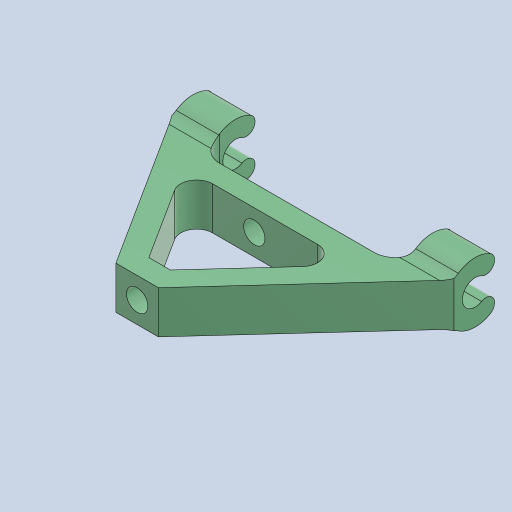
# Autodesk Inventor part: GearBase
Saved by Autodesk Inventor 2023 (Build 270158000, 158)
## iProperties
Created: 2022-06-15
Part Number: GearBase
Material: ABS プラスチック
Document SubType Name: Modeling
Designer: legot
Density: 1.06 g/cm^3
Appearance: 滑らか - 白
Mass: 0.555429 g
Surface Area: 7.58105 cm^2
Volume: 0.52399 cm^3
Author: legot
Autodesk Inventor part; units mm, degrees
ref_plane "YZ Plane" through (0, 0, 0) normal (1, 0, 0) x (0, 1, 0)
ref_plane "XZ Plane" through (0, 0, 0) normal (0, 1, 0) x (-1, 0, 0)
ref_plane "XY Plane" through (0, 0, 0) normal (0, 0, 1) x (1, 0, 0)
sketch "スケッチ1" plane through (0, 0, 0) normal (0, 1, 0) x (-1, 0, 0)
  line L0 (13.25, -2) -> (-13.25, -2)
  line L1 (-13.25, -2) -> (-13.25, 2)
  line L2 (13.25, 2) -> (13.25, -2)
  line L3 (13.25, 2) -> (4, 16.5)
  line L4 (4, 16.5) -> (0, 16.5)
  line L5 (0, 16.5) -> (-13.25, 2)
  line L6 (9.25, 3.5) -> (-9.25, 3.5)
  line L7 (9.25, 3.5) -> (9.25, -2)
  line L8 (-9.25, 3.5) -> (-9.25, -2)
  point P0 (0, 0)
  point P1 (13.25, 0)
  point P2 (0, -2)
  point P3 (2, 16.5)
  dimension "d1" = 4
  dimension "d2" = 4
  dimension "d3" = 16.5
  dimension "d19" = 3.5
  dimension "d32" = 4
  dimension "d33" = 26.5
  dimension "d34" = 4
  dimension "d36" = 4
  dimension "d37" = 2
  constraints: 18 end point, 3 horizontal, 3 midpoint, 2 parallel, 2 perpendicular, 2 point on line, 1 horizontal alignment, 1 vertical alignment
  measures "d1" distance of L2.start L0.start
  measures "d2" distance of L3.end L4.end
  measures "d3" distance from line of point (0, 0) L4
  measures "d19" distance from line of L6 point (0, 0)
  measures "d32" distance between parallel lines of L8 L1
  measures "d33" distance of L0.start L0.end
  measures "d34" distance between parallel lines of L2 L7
  measures "d36" distance of L0.end L1.end
  measures "d37" horizontal distance of point (0, -2) point (2, 16.5)
extrude "押し出し1" add sketch "スケッチ1" along normal mid plane 4 contours L0 L7 L6 L8 L1 L5 L4 L3 L2
sketch "スケッチ3" plane through (-4, 2, 16.5) normal (0, 0, 1) x (1, 0, 0)
  line L0 (0, 0) -> (4, 0) projected
  line L1 (0, -4) -> (0, 0) projected
  point P0 (4, -2)
  point P1 (2, -2)
  point P2 (0, -2)
  point P3 (2, 0)
  constraints: 2 midpoint, 1 horizontal alignment, 1 vertical alignment
hole "穴1" at (-2, 0, 16.5) direction (0, 0, -1) diameter 2 end through all
sketch "スケッチ4" plane through (13.25, -2, -2) normal (1, 0, 0) x (0, 0, -1)
  line L0 (0, 4) -> (0, 0) projected
  line L1 (-4, 0) -> (-4, 4) projected
  line L2 (0, 0) -> (-4, 0) projected
  circle A0 centre (-2, 2) radius 1.2
  line L3 (-4, 4) -> (0, 4) projected
  arc A1 (-4, 0) -> (-4, 4) centre (-2, 2) ccw
  circle A2 centre (-0.9929, 3.7444) radius 0.8142
  circle A3 centre (-0.9929, 0.2556) radius 0.8142
  line L4 (-0.9929, 3.7444) -> (-2, 2) construction
  line L5 (-2, 2) -> (-0.9929, 0.2556) construction
  line L6 (-0.9929, 1.0699) -> (-0.9929, 2.9301) construction
  line L7 (0, 2.2089) -> (-0.9929, 3.7444) construction
  point P0 (-2, 2)
  point P1 (-1.4, 3.0392)
  point P2 (-1.4, 0.9608)
  point P3 (-0.2199, 0)
  point P4 (-0.2199, 4)
  point P5 (-0.5858, 4.4495)
  point P6 (-0.5858, -0.4495)
  dimension "d22" = 1.6284
  dimension "d20" = 2.4
  dimension "d21" = 120
  dimension "d23" = 1.8603
  constraints: 10 end point, 3 point on circle, 3 point on line, 2 centre point, 2 coincident, 1 vertical alignment, 10 other
  measures "d20" diameter of A0
  measures "d21" angle of L5 L4
  measures "d23" distance of L6.start L6.end
extrude "押し出し3" add sketch "スケッチ4" against normal up to surface (4 mm away)
extrude "押し出し4" cut sketch "スケッチ4" against normal up to surface (4 mm away) contours A1 L0 | L0 L2 A3 A0 A2 L3 | L3 A2 A1 | A1 A3 L2 | A0 picked at (-0.1339, 4.0556) picked at (-0.1339, -0.0556)
mirror "ミラー1" about plane through (0, 0, 0) normal (1, 0, 0) of "押し出し3", "押し出し4"
sketch "スケッチ5" plane through (0, 2, 0) normal (0, 1, 0) x (1, 0, 0)
  line L0 (-13.25, -2) -> (-4, -16.5) projected
  line L1 (-4, -16.5) -> (0, -16.5) projected
  line L2 (0, -16.5) -> (13.25, -2) projected
  line L3 (9.25, -3.5) -> (-9.25, -3.5) projected
  line L4 (-2.9036, -14.5) -> (-8.6449, -5.5)
  line L5 (7.3425, -5.5) -> (-0.8817, -14.5)
  line L6 (-0.8817, -14.5) -> (-2.9036, -14.5)
  line L7 (-8.6449, -5.5) -> (7.3425, -5.5)
  point P0 (0, 0)
  dimension "d38" = 2
  dimension "d40" = 2
  dimension "d41" = 2
  constraints: 9 end point, 1 horizontal, 1 parallel, 1 other
  measures "d38" distance between parallel lines of L2 L5
  measures "d40" distance between parallel lines of L0 L4
  measures "d41" distance between parallel lines of L3 L7
extrude "押し出し5" cut sketch "スケッチ5" against normal through all
fillet "フィレット4" radius 1.5 2 edges at (-8.6449, 0, 5.5) (7.3425, 0, 5.5)
fillet "フィレット5" radius 2 6 edges at (9.25, 0, 3.5) (-9.25, 0, 3.5) (-11.25, 2, 2) (11.25, 2, 2) (11.25, -2, 2) (-11.25, -2, 2)
equation "\"d34\" = d32"
equation "\"d36\" = d1"
equation "\"d37\" = 0.5 * d32"
equation "\"d40\" = d38"
equation "\"d41\" = d38"
